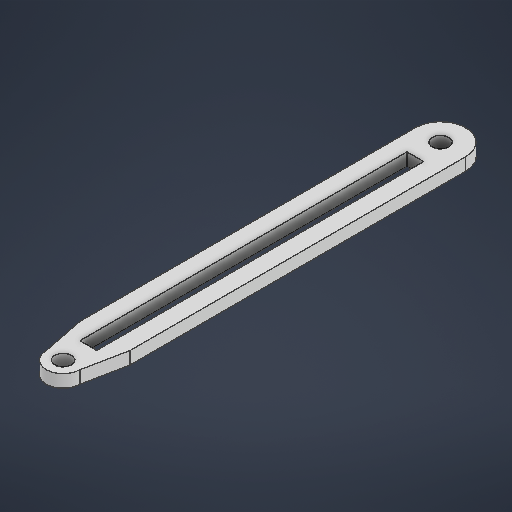
# Autodesk Inventor part: measuring_slider1_lid
Saved by Autodesk Inventor 2026.1 (Build 301233000, 233)
## iProperties
Created: 2025-12-25
Part Number: measuring_slider1_lid
Material: Generic
Document SubType Name: Modeling
Designer: emanuel
Density: 1 g/cm^3
Appearance: Default
Author: emanuel
Autodesk Inventor part; units mm, degrees
ref_plane "YZ Plane" through (0, 0, 0) normal (1, 0, 0) x (0, 1, 0)
ref_plane "XZ Plane" through (0, 0, 0) normal (0, 1, 0) x (-1, 0, 0)
ref_plane "XY Plane" through (0, 0, 0) normal (0, 0, 1) x (1, 0, 0)
sketch "Sketch1" plane through (0, 0, 0) normal (0, 1, 0) x (-1, 0, 0)
  circle A0 centre (0, 0) radius 1
  line L0 (0, 0) -> (0, -45)
  circle A1 centre (0, -45) radius 1
  circle A2 centre (0, -45) radius 3
  circle A3 centre (0, 0) radius 2
  line L1 (3, -45) -> (-3, -45)
  line L2 (-3, -45) -> (-3, -5)
  line L3 (-3, -5) -> (3, -5)
  line L4 (3, -5) -> (3, -45)
  line L5 (2, 0) -> (3, -5)
  line L6 (-2, 0) -> (-3, -5)
  dimension "d2" = 6
  dimension "d0" = 2
  dimension "d1" = 45
  dimension "d3" = 4
  dimension "d4" = 40
  constraints: 14 end point, 4 coincident, 3 centre point, 2 parallel, 2 point on circle, 1 horizontal, 1 perpendicular, 1 vertical, 3 other
  measures "d0" diameter of A0
  measures "d1" distance of L0.start L0.end
  measures "d3" diameter of A3
  measures "d4" distance of L1.end L2.end
extrude "Extrusion1" add sketch "Sketch1" along normal blind 1.5 contours A3 L5 L3 L0 | L0 L3 L6 A3 | A3 | L3 L4 A2 L0 | L0 A2 L2 L3 | A2 L1 A1 L0 | L0 A1 L1 A2 | A2 L1 A1
sketch "Sketch2" plane through (0, 1.5, 0) normal (0, 1, 0) x (1, 0, 0)
  circle A0 centre (0, 45) radius 1 projected
  line L0 (0, 45) -> (0, 42)
  circle A1 centre (0, 0) radius 1 projected
  line L1 (0, 0) -> (0, 3)
  line L2 (0, 3) -> (1, 3)
  line L3 (1, 3) -> (-1, 3)
  line L4 (-1, 3) -> (-1, 42)
  line L5 (-1, 42) -> (1, 42)
  line L6 (1, 42) -> (1, 3)
  dimension "d7" = 3
  dimension "d8" = 3
  dimension "d9" = 1
  dimension "d10" = 2
  constraints: 14 end point, 2 horizontal, 2 parallel, 2 vertical, 1 perpendicular
  measures "d7" distance of L0.start L0.end
  measures "d8" distance of L1.start L1.end
  measures "d9" distance of L1.end L2.end
  measures "d10" distance of L4.end L5.end
extrude "Extrusion2" cut sketch "Sketch2" against normal blind 1.5 contours L3 L4 L5 L6 L2
body "Solid1"
